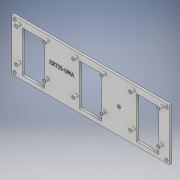
# Autodesk Inventor part: ClusterLayer3-2
Saved by Autodesk Inventor 2019 (Build 230136000, 136)
## iProperties
Created: 2019-02-04
Part Number: ClusterLayer3-2
Material: Genérico
Document SubType Name: Modeling
Designer: LuisAlonso
Density: 1 g/cm^3
Appearance: Valor por defecto
Author: LuisAlonso
Autodesk Inventor part; units mm, degrees
ref_plane "YZ Plane" through (0, 0, 0) normal (1, 0, 0) x (0, 1, 0)
ref_plane "XZ Plane" through (0, 0, 0) normal (0, 1, 0) x (-1, 0, 0)
ref_plane "XY Plane" through (0, 0, 0) normal (0, 0, 1) x (1, 0, 0)
sketch "Boceto1" plane through (0, 0, 0) normal (0, 0, 1) x (1, 0, 0)
  line L0 (0, 0) -> (275, 0)
  line L1 (275, 0) -> (275, -90)
  line L2 (275, -90) -> (0, -90)
  line L3 (0, -90) -> (0, 0)
  dimension "d0" = 275
  dimension "d1" = 90
  constraints: 8 end point, 2 perpendicular, 1 horizontal, 1 vertical
  measures "d0" distance of L0.start L0.end
  measures "d1" distance of L0.end L1.end
extrude "Extrusión1" add sketch "Boceto1" along normal blind 4
sketch "Boceto8" plane through (0, 0, 4) normal (0, 0, 1) x (1, 0, 0)
  line L0 (275, 0) -> (0, 0) projected
  line L1 (0, 0) -> (5, 0)
  line L2 (5, 0) -> (5, -5)
  circle A0 centre (5, -5) radius 1.6
  line L3 (0, 0) -> (0, -90) projected
  line L4 (0, -90) -> (5, -90)
  line L5 (5, -90) -> (5, -85)
  circle A1 centre (5, -85) radius 1.6
  line L6 (0, -90) -> (275, -90) projected
  line L7 (275, -90) -> (270, -90)
  line L8 (270, -90) -> (270, -85)
  circle A2 centre (270, -85) radius 1.6
  line L9 (275, 0) -> (270, 0)
  line L10 (270, 0) -> (270, -5)
  circle A3 centre (270, -5) radius 1.6
  dimension "d127" = 5
  dimension "d128" = 5
  dimension "d129" = 3.2
  dimension "d130" = 5
  dimension "d131" = 5
  dimension "d132" = 3.2
  dimension "d133" = 5
  dimension "d134" = 5
  dimension "d135" = 3.2
  dimension "d136" = 5
  dimension "d137" = 5
  dimension "d138" = 3.2
  constraints: 16 end point, 4 centre point, 4 coincident, 4 perpendicular, 3 point on line, 1 horizontal
  measures "d127" distance of L0.end L1.end
  measures "d128" distance of L1.end L2.end
  measures "d129" diameter of A0
  measures "d130" distance of L3.end L4.end
  measures "d131" distance of L4.end L5.end
  measures "d132" diameter of A1
  measures "d133" distance of L6.end L7.end
  measures "d134" distance of L7.end L8.end
  measures "d135" diameter of A2
  measures "d136" distance of L0.start L9.end
  measures "d137" distance of L9.end L10.end
  measures "d138" diameter of A3
extrude "Extrusión7" cut sketch "Boceto8" against normal blind 15
sketch "Boceto9" plane through (0, 0, 4) normal (0, 0, 1) x (1, 0, 0)
  line L0 (0, 0) -> (13.5, 0)
  line L1 (0, 0) -> (275, 0) projected
  line L2 (13.5, 0) -> (13.5, -8)
  circle A0 centre (13.5, -8) radius 1.5
  line L3 (13.5, -8) -> (62.5, -8)
  line L4 (13.5, -8) -> (13.5, -66)
  line L5 (62.5, -8) -> (62.5, -66)
  circle A1 centre (62.5, -8) radius 1.5
  circle A2 centre (62.5, -66) radius 1.5
  circle A3 centre (13.5, -66) radius 1.5
  dimension "d141" = 13.5
  dimension "d142" = 8
  dimension "d143" = 3
  dimension "d144" = 49
  dimension "d145" = 58
  dimension "d146" = 58
  dimension "d147" = 3
  dimension "d148" = 3
  dimension "d149" = 3
  constraints: 10 end point, 4 centre point, 4 coincident, 2 vertical, 1 horizontal, 1 perpendicular, 1 point on line
  measures "d141" distance of L0.start L0.end
  measures "d142" distance of L0.end L2.end
  measures "d143" diameter of A0
  measures "d144" distance of L3.start L3.end
  measures "d145" distance of L3.start L4.end
  measures "d146" distance of L3.end L5.end
  measures "d147" diameter of A1
  measures "d148" diameter of A2
  measures "d149" diameter of A3
extrude "Extrusión8" cut sketch "Boceto9" against normal blind 15
sketch "Boceto10" plane through (0, 0, 4) normal (0, 0, 1) x (1, 0, 0)
  line L0 (0, 0) -> (275, 0) projected
  line L1 (275, 0) -> (261.5, 0)
  line L2 (261.5, 0) -> (261.5, -8)
  circle A0 centre (261.5, -8) radius 1.5
  line L3 (261.5, -8) -> (261.5, -66)
  line L4 (261.5, -66) -> (212.5, -66)
  line L5 (212.5, -66) -> (212.5, -8)
  circle A1 centre (212.5, -8) radius 1.5
  circle A2 centre (212.5, -66) radius 1.5
  circle A3 centre (261.5, -66) radius 1.5
  dimension "d152" = 13.5
  dimension "d153" = 8
  dimension "d154" = 3
  dimension "d155" = 58
  dimension "d156" = 49
  dimension "d157" = 3
  dimension "d158" = 3
  dimension "d159" = 3
  constraints: 10 end point, 4 centre point, 4 coincident, 3 perpendicular, 1 point on line, 1 vertical
  measures "d152" distance of L0.end L1.end
  measures "d153" distance of L1.end L2.end
  measures "d154" diameter of A0
  measures "d155" distance of L3.start L3.end
  measures "d156" distance of L3.end L4.end
  measures "d157" diameter of A1
  measures "d158" diameter of A2
  measures "d159" diameter of A3
extrude "Extrusión9" cut sketch "Boceto10" against normal blind 15
sketch "Boceto11" plane through (0, 0, 4) normal (0, 0, 1) x (1, 0, 0)
  line L0 (0, 0) -> (113, 0)
  line L1 (0, 0) -> (275, 0) projected
  line L2 (113, 0) -> (113, -8)
  circle A0 centre (113, -8) radius 1.5
  line L3 (113, -8) -> (162, -8)
  line L4 (162, -8) -> (162, -66)
  line L5 (162, -66) -> (113, -66)
  circle A1 centre (113, -66) radius 1.5
  circle A2 centre (162, -66) radius 1.5
  circle A3 centre (162, -8) radius 1.5
  dimension "d162" = 113
  dimension "d163" = 8
  dimension "d164" = 3
  dimension "d165" = 49
  dimension "d166" = 58
  dimension "d167" = 3
  dimension "d168" = 3
  dimension "d169" = 3
  constraints: 10 end point, 4 centre point, 4 coincident, 3 perpendicular, 1 horizontal, 1 point on line
  measures "d162" distance of L0.start L0.end
  measures "d163" distance of L0.end L2.end
  measures "d164" diameter of A0
  measures "d165" distance of L3.start L3.end
  measures "d166" distance of L3.end L4.end
  measures "d167" diameter of A1
  measures "d168" diameter of A2
  measures "d169" diameter of A3
extrude "Extrusión10" cut sketch "Boceto11" against normal blind 15
sketch "Boceto12" plane through (0, 0, 4) normal (0, 0, 1) x (1, 0, 0)
  line L0 (275, -90) -> (0, -90) projected
  line L1 (275, -90) -> (187.25, -90)
  line L2 (187.25, -90) -> (187.25, -46)
  circle A0 centre (187.25, -46) radius 1.6
  point P0 (0, 0)
  dimension "d172" = 87.75
  dimension "d173" = 44
  dimension "d174" = 3.2
  constraints: 4 end point, 1 centre point, 1 coincident, 1 point on line, 1 vertical
  measures "d172" distance of L0.start L1.end
  measures "d173" distance of L1.end L2.end
  measures "d174" diameter of A0
extrude "Extrusión11" cut sketch "Boceto12" against normal blind 15
sketch "Boceto13" plane through (0, 0, 4) normal (0, 0, 1) x (1, 0, 0)
  line L0 (0, -90) -> (0, 0) projected
  line L1 (0, 0) -> (18.5, 0)
  line L2 (0, 0) -> (275, 0) projected
  line L3 (18.5, 0) -> (18.5, -11)
  line L4 (18.5, -11) -> (57.5, -11)
  line L5 (57.5, -11) -> (57.5, -83)
  line L6 (57.5, -83) -> (18.5, -83)
  line L7 (18.5, -83) -> (18.5, -11)
  dimension "d177" = 18.5
  dimension "d178" = 11
  dimension "d179" = 39
  dimension "d180" = 72
  dimension "d181" = 39
  constraints: 12 end point, 2 horizontal, 2 perpendicular, 1 point on line
  measures "d177" distance of L0.end L1.end
  measures "d178" distance of L1.end L3.end
  measures "d179" distance of L3.end L4.end
  measures "d180" distance of L4.end L5.end
  measures "d181" distance of L5.end L6.end
extrude "Extrusión12" cut sketch "Boceto13" against normal blind 15
sketch "Boceto14" plane through (0, 0, 4) normal (0, 0, 1) x (1, 0, 0)
  line L0 (275, 0) -> (275, -90) projected
  line L1 (275, 0) -> (256.5, 0)
  line L2 (0, 0) -> (275, 0) projected
  line L3 (256.5, 0) -> (256.5, -11)
  line L4 (256.5, -11) -> (217.5, -11)
  line L5 (217.5, -11) -> (217.5, -83)
  line L6 (217.5, -83) -> (256.5, -83)
  line L7 (256.5, -83) -> (256.5, -11)
  dimension "d184" = 18.5
  dimension "d185" = 11
  dimension "d186" = 39
  dimension "d187" = 72
  dimension "d188" = 39
  constraints: 12 end point, 3 perpendicular, 2 point on line
  measures "d184" distance of L0.start L1.end
  measures "d185" distance of L1.end L3.end
  measures "d186" distance of L3.end L4.end
  measures "d187" distance of L4.end L5.end
  measures "d188" distance of L5.end L6.end
extrude "Extrusión13" cut sketch "Boceto14" against normal blind 15
sketch "Boceto15" plane through (0, 0, 4) normal (0, 0, 1) x (1, 0, 0)
  line L0 (0, 0) -> (275, 0) projected
  line L1 (0, 0) -> (118, 0)
  line L2 (118, 0) -> (118, -11)
  line L3 (118, -11) -> (157, -11)
  line L4 (157, -11) -> (157, -83)
  line L5 (157, -83) -> (118, -83)
  line L6 (118, -83) -> (118, -11)
  dimension "d191" = 118
  dimension "d192" = 11
  dimension "d193" = 39
  dimension "d194" = 72
  dimension "d195" = 39
  constraints: 12 end point, 2 horizontal, 2 perpendicular, 1 point on line
  measures "d191" distance of L0.start L1.end
  measures "d192" distance of L1.end L2.end
  measures "d193" distance of L2.end L3.end
  measures "d194" distance of L3.end L4.end
  measures "d195" distance of L4.end L5.end
extrude "Extrusión14" cut sketch "Boceto15" against normal blind 15
sketch "Boceto17" plane through (0, 0, 4) normal (0, 0, 1) x (1, 0, 0)
  circle A0 centre (5, -5) radius 1.6 projected
  circle A1 centre (5, -5) radius 3
  circle A2 centre (13.5, -8) radius 1.5 projected
  circle A3 centre (13.5, -8) radius 3
  circle A4 centre (62.5, -8) radius 1.5 projected
  circle A5 centre (62.5, -8) radius 3
  circle A6 centre (62.5, -66) radius 1.5 projected
  circle A7 centre (62.5, -66) radius 3
  circle A8 centre (13.5, -66) radius 1.5 projected
  circle A9 centre (13.5, -66) radius 3
  circle A10 centre (5, -85) radius 1.6 projected
  circle A11 centre (5, -85) radius 3
  circle A12 centre (113, -8) radius 1.5 projected
  circle A13 centre (113, -8) radius 3
  circle A14 centre (162, -8) radius 1.5 projected
  circle A15 centre (162, -8) radius 3
  circle A16 centre (113, -66) radius 1.5 projected
  circle A17 centre (113, -66) radius 3
  circle A18 centre (162, -66) radius 1.5 projected
  circle A19 centre (162, -66) radius 3
  circle A20 centre (187.25, -46) radius 1.6 projected
  circle A21 centre (187.25, -46) radius 3
  circle A22 centre (212.5, -8) radius 1.5 projected
  circle A23 centre (212.5, -8) radius 3
  circle A24 centre (212.5, -66) radius 1.5 projected
  circle A25 centre (212.5, -66) radius 3
  circle A26 centre (261.5, -8) radius 1.5 projected
  circle A27 centre (261.5, -8) radius 3
  circle A28 centre (270, -5) radius 1.6 projected
  circle A29 centre (270, -5) radius 3
  circle A30 centre (261.5, -66) radius 1.5 projected
  circle A31 centre (261.5, -66) radius 3
  circle A32 centre (270, -85) radius 1.6 projected
  circle A33 centre (270, -85) radius 3
  circle A34 centre (62.5, -66) radius 2
  circle A35 centre (113, -8) radius 2
  circle A36 centre (162, -8) radius 2
  circle A37 centre (212.5, -8) radius 2
  circle A38 centre (212.5, -66) radius 2
  circle A39 centre (162, -66) radius 2
  circle A40 centre (113, -66) radius 2
  circle A41 centre (261.5, -8) radius 2
  circle A42 centre (261.5, -66) radius 2
  circle A43 centre (62.5, -8) radius 1.5 projected
  circle A44 centre (62.5, -8) radius 2
  circle A45 centre (13.5, -8) radius 2
  circle A46 centre (13.5, -66) radius 2
  point P0 (0, 0)
  dimension "d198" = 6
  dimension "d199" = 6
  dimension "d200" = 6
  dimension "d201" = 6
  dimension "d202" = 6
  dimension "d203" = 6
  dimension "d204" = 6
  dimension "d205" = 6
  dimension "d206" = 6
  dimension "d207" = 6
  dimension "d208" = 6
  dimension "d209" = 6
  dimension "d210" = 6
  dimension "d211" = 6
  dimension "d212" = 6
  dimension "d213" = 6
  dimension "d214" = 6
  dimension "d232" = 4
  dimension "d233" = 4
  dimension "d234" = 4
  dimension "d235" = 4
  dimension "d236" = 4
  dimension "d237" = 4
  dimension "d238" = 4
  dimension "d239" = 4
  dimension "d240" = 4
  dimension "d241" = 4
  dimension "d242" = 4
  dimension "d243" = 4
  constraints: 29 centre point, 29 coincident
  measures "d198" diameter of A1
  measures "d199" diameter of A3
  measures "d200" diameter of A5
  measures "d201" diameter of A7
  measures "d202" diameter of A9
  measures "d203" diameter of A11
  measures "d204" diameter of A13
  measures "d205" diameter of A15
  measures "d206" diameter of A17
  measures "d207" diameter of A19
  measures "d208" diameter of A21
  measures "d209" diameter of A23
  measures "d210" diameter of A25
  measures "d211" diameter of A27
  measures "d212" diameter of A29
  measures "d213" diameter of A31
  measures "d214" diameter of A33
  measures "d232" diameter of A34
  measures "d233" diameter of A35
  measures "d234" diameter of A36
  measures "d235" diameter of A37
  measures "d236" diameter of A38
  measures "d237" diameter of A39
  measures "d238" diameter of A40
  measures "d239" diameter of A41
  measures "d240" diameter of A42
  measures "d241" diameter of A44
  measures "d242" diameter of A45
  measures "d243" diameter of A46
sketch "Boceto24" plane through (0, 0, 4) normal (0, 0, 1) x (1, 0, 0)
  line L0 (65.986, -35.14) -> (108.7206, -35.14) construction
  line L1 (108.7206, -35.14) -> (108.7206, -41.4773) construction
  line L2 (108.7206, -41.4773) -> (65.986, -41.4773) construction
  line L3 (65.986, -41.4773) -> (65.986, -35.14) construction
  line L4 (66.6039, -41.3488) -> (66.6039, -35.2488)
  line L5 (66.6039, -35.2488) -> (70.4201, -35.2488)
  line L6 (70.4201, -35.2488) -> (70.4201, -35.9705)
  line L7 (70.4201, -35.9705) -> (67.4146, -35.9705)
  line L8 (67.4146, -35.9705) -> (67.4146, -37.6413)
  line L9 (67.4146, -37.6413) -> (70.2174, -37.6413)
  line L10 (70.2174, -37.6413) -> (70.2174, -38.363)
  line L11 (70.2174, -38.363) -> (67.4146, -38.363)
  line L12 (67.4146, -38.363) -> (67.4146, -40.6271)
  line L13 (67.4146, -40.6271) -> (70.4201, -40.6271)
  line L14 (70.4201, -40.6271) -> (70.4201, -41.3488)
  line L15 (70.4201, -41.3488) -> (66.6039, -41.3488)
  line L16 (76.0307, -41.3488) -> (74.9778, -41.3488)
  line L17 (74.9778, -41.3488) -> (73.0499, -38.9216)
  line L18 (73.0499, -38.9216) -> (72.1206, -38.9216)
  line L19 (72.1206, -38.9216) -> (72.1206, -41.3488)
  line L20 (72.1206, -41.3488) -> (71.3099, -41.3488)
  line L21 (71.3099, -41.3488) -> (71.3099, -35.2488)
  line L22 (71.3099, -35.2488) -> (72.8819, -35.2488)
  spline S0 degree 2 poles (72.8819, -35.2488) (73.4058, -35.2488) (74.1127, -35.3625) (74.434, -35.5701) knots 0 0 0 1 2 2 2
  spline S1 degree 2 poles (74.434, -35.5701) (74.7554, -35.7777) (75.1261, -36.4253) (75.1261, -36.9048) knots 0 0 0 1 2 2 2
  spline S2 degree 2 poles (75.1261, -36.9048) (75.1261, -37.5721) (74.4439, -38.4767) (73.8606, -38.6942) knots 0 0 0 1 2 2 2
  line L23 (73.8606, -38.6942) -> (76.0307, -41.3488)
  spline S3 degree 2 poles (74.2808, -36.969) (74.2808, -36.7021) (74.093, -36.2918) (73.8952, -36.1583) knots 0 0 0 1 2 2 2
  spline S4 degree 2 poles (73.8952, -36.1583) (73.7222, -36.0446) (73.2625, -35.9507) (72.9263, -35.9507) knots 0 0 0 1 2 2 2
  line L24 (72.9263, -35.9507) -> (72.1206, -35.9507)
  line L25 (72.1206, -35.9507) -> (72.1206, -38.2444)
  line L26 (72.1206, -38.2444) -> (72.8324, -38.2444)
  spline S5 degree 2 poles (72.8324, -38.2444) (73.1834, -38.2444) (73.742, -38.1208) (73.9348, -37.928) knots 0 0 0 1 2 2 2
  spline S6 degree 2 poles (73.9348, -37.928) (74.1127, -37.76) (74.2808, -37.2854) (74.2808, -36.969) knots 0 0 0 1 2 2 2
  line L27 (77.9388, -41.3488) -> (77.9388, -35.9705)
  line L28 (77.9388, -35.9705) -> (75.8923, -35.9705)
  line L29 (75.8923, -35.9705) -> (75.8923, -35.2488)
  line L30 (75.8923, -35.2488) -> (80.796, -35.2488)
  line L31 (80.796, -35.2488) -> (80.796, -35.9705)
  line L32 (80.796, -35.9705) -> (78.7495, -35.9705)
  line L33 (78.7495, -35.9705) -> (78.7495, -41.3488)
  line L34 (78.7495, -41.3488) -> (77.9388, -41.3488)
  line L35 (83.5396, -41.3488) -> (81.1767, -41.3488)
  line L36 (81.1767, -41.3488) -> (81.1767, -40.7259)
  line L37 (81.1767, -40.7259) -> (81.9528, -40.7259)
  line L38 (81.9528, -40.7259) -> (81.9528, -35.8716)
  line L39 (81.9528, -35.8716) -> (81.1767, -35.8716)
  line L40 (81.1767, -35.8716) -> (81.1767, -35.2488)
  line L41 (81.1767, -35.2488) -> (83.5396, -35.2488)
  line L42 (83.5396, -35.2488) -> (83.5396, -35.8716)
  line L43 (83.5396, -35.8716) -> (82.7635, -35.8716)
  line L44 (82.7635, -35.8716) -> (82.7635, -40.7259)
  line L45 (82.7635, -40.7259) -> (83.5396, -40.7259)
  line L46 (83.5396, -40.7259) -> (83.5396, -41.3488)
  spline S7 degree 2 poles (86.2435, -41.4575) (85.5811, -41.4575) (84.6518, -41.1807) (84.2415, -40.983) knots 0 0 0 1 2 2 2
  line L47 (84.2415, -40.983) -> (84.2415, -39.9647)
  line L48 (84.2415, -39.9647) -> (84.3008, -39.9647)
  spline S8 degree 2 poles (84.3008, -39.9647) (84.7012, -40.3404) (85.7146, -40.7556) (86.1842, -40.7556) knots 0 0 0 1 2 2 2
  spline S9 degree 2 poles (86.1842, -40.7556) (86.8565, -40.7556) (87.5436, -40.197) (87.5436, -39.7373) knots 0 0 0 1 2 2 2
  spline S10 degree 2 poles (87.5436, -39.7373) (87.5436, -39.3715) (87.1828, -38.9167) (86.7922, -38.803) knots 0 0 0 1 2 2 2
  spline S11 degree 2 poles (86.7922, -38.803) (86.5105, -38.7239) (86.0409, -38.6151) (85.6899, -38.5262) knots 0 0 0 1 2 2 2
  spline S12 degree 2 poles (85.6899, -38.5262) (85.3735, -38.4421) (84.8742, -38.19) (84.6815, -37.9874) knots 0 0 0 1 2 2 2
  spline S13 degree 2 poles (84.6815, -37.9874) (84.4936, -37.7847) (84.286, -37.2409) (84.286, -36.885) knots 0 0 0 1 2 2 2
  spline S14 degree 2 poles (84.286, -36.885) (84.286, -36.1435) (85.4427, -35.14) (86.3375, -35.14) knots 0 0 0 1 2 2 2
  spline S15 degree 2 poles (86.3375, -35.14) (86.8516, -35.14) (87.7611, -35.3427) (88.1516, -35.5355) knots 0 0 0 1 2 2 2
  line L49 (88.1516, -35.5355) -> (88.1516, -36.5044)
  line L50 (88.1516, -36.5044) -> (88.0923, -36.5044)
  spline S16 degree 2 poles (88.0923, -36.5044) (87.8007, -36.2374) (86.8911, -35.842) (86.3918, -35.842) knots 0 0 0 1 2 2 2
  spline S17 degree 2 poles (86.3918, -35.842) (85.8283, -35.842) (85.1313, -36.3709) (85.1313, -36.801) knots 0 0 0 1 2 2 2
  spline S18 degree 2 poles (85.1313, -36.801) (85.1313, -37.1865) (85.5416, -37.6463) (85.9272, -37.7501) knots 0 0 0 1 2 2 2
  spline S19 degree 2 poles (85.9272, -37.7501) (86.1842, -37.8193) (86.9306, -37.9972) (87.1778, -38.0714) knots 0 0 0 1 2 2 2
  spline S20 degree 2 poles (87.1778, -38.0714) (87.8056, -38.2642) (88.3889, -39.0403) (88.3889, -39.6087) knots 0 0 0 1 2 2 2
  spline S21 degree 2 poles (88.3889, -39.6087) (88.3889, -39.9696) (88.0973, -40.6617) (87.8353, -40.9039) knots 0 0 0 1 2 2 2
  spline S22 degree 2 poles (87.8353, -40.9039) (87.5436, -41.1708) (86.8021, -41.4575) (86.2435, -41.4575) knots 0 0 0 1 2 2 2
  line L51 (91.2758, -39.0502) -> (88.9673, -39.0502)
  line L52 (88.9673, -39.0502) -> (88.9673, -38.3087)
  line L53 (88.9673, -38.3087) -> (91.2758, -38.3087)
  line L54 (91.2758, -38.3087) -> (91.2758, -39.0502)
  spline S23 degree 2 poles (94.39, -41.4773) (93.8512, -41.4773) (93.0504, -41.1955) (92.7687, -40.9138) knots 0 0 0 1 2 2 2
  spline S24 degree 2 poles (92.7687, -40.9138) (92.4473, -40.5974) (92.1853, -39.7076) (92.1853, -39.0551) knots 0 0 0 1 2 2 2
  line L55 (92.1853, -39.0551) -> (92.1853, -35.2488)
  line L56 (92.1853, -35.2488) -> (92.996, -35.2488)
  line L57 (92.996, -35.2488) -> (92.996, -39.0551)
  spline S25 degree 2 poles (92.996, -39.0551) (92.996, -39.4802) (93.1048, -40.0536) (93.258, -40.286) knots 0 0 0 1 2 2 2
  spline S26 degree 2 poles (93.258, -40.286) (93.4212, -40.5331) (93.9847, -40.7852) (94.39, -40.7852) knots 0 0 0 1 2 2 2
  spline S27 degree 2 poles (94.39, -40.7852) (94.7707, -40.7852) (95.3639, -40.5331) (95.527, -40.286) knots 0 0 0 1 2 2 2
  spline S28 degree 2 poles (95.527, -40.286) (95.6802, -40.0536) (95.789, -39.4852) (95.789, -39.0749) knots 0 0 0 1 2 2 2
  line L58 (95.789, -39.0749) -> (95.789, -35.2488)
  line L59 (95.789, -35.2488) -> (96.5997, -35.2488)
  line L60 (96.5997, -35.2488) -> (96.5997, -39.0551)
  spline S29 degree 2 poles (96.5997, -39.0551) (96.5997, -39.6928) (96.3426, -40.6023) (96.0164, -40.9138) knots 0 0 0 1 2 2 2
  spline S30 degree 2 poles (96.0164, -40.9138) (95.7247, -41.2005) (94.9536, -41.4773) (94.39, -41.4773) knots 0 0 0 1 2 2 2
  line L61 (102.9913, -41.3488) -> (102.1806, -41.3488)
  line L62 (102.1806, -41.3488) -> (102.1806, -36.0941)
  line L63 (102.1806, -36.0941) -> (100.5889, -39.6681)
  line L64 (100.5889, -39.6681) -> (100.0946, -39.6681)
  line L65 (100.0946, -39.6681) -> (98.5177, -36.0941)
  line L66 (98.5177, -36.0941) -> (98.5177, -41.3488)
  line L67 (98.5177, -41.3488) -> (97.7614, -41.3488)
  line L68 (97.7614, -41.3488) -> (97.7614, -35.2488)
  line L69 (97.7614, -35.2488) -> (98.8687, -35.2488)
  line L70 (98.8687, -35.2488) -> (100.3912, -38.6448)
  line L71 (100.3912, -38.6448) -> (101.8643, -35.2488)
  line L72 (101.8643, -35.2488) -> (102.9913, -35.2488)
  line L73 (102.9913, -35.2488) -> (102.9913, -41.3488)
  line L74 (103.5697, -41.3488) -> (105.6261, -35.2488)
  line L75 (105.6261, -35.2488) -> (106.6246, -35.2488)
  line L76 (106.6246, -35.2488) -> (108.681, -41.3488)
  line L77 (108.681, -41.3488) -> (107.8259, -41.3488)
  line L78 (107.8259, -41.3488) -> (107.2722, -39.6433)
  line L79 (107.2722, -39.6433) -> (104.9439, -39.6433)
  line L80 (104.9439, -39.6433) -> (104.3903, -41.3488)
  line L81 (104.3903, -41.3488) -> (103.5697, -41.3488)
  line L82 (107.0498, -38.9513) -> (106.1056, -36.0792)
  line L83 (106.1056, -36.0792) -> (105.1664, -38.9513)
  line L84 (105.1664, -38.9513) -> (107.0498, -38.9513)
  point P0 (0, 0)
  constraints: 2 other
extrude "Extrusión17" cut sketch "Boceto24" against normal blind 10
sketch "Boceto26" plane through (0, 0, 4) normal (0, 0, 1) x (1, 0, 0)
  circle A0 centre (5, -5) radius 1.6 projected
  circle A1 centre (5, -5) radius 3
  circle A2 centre (270, -85) radius 1.6 projected
  circle A3 centre (270, -85) radius 3
  circle A4 centre (270, -5) radius 1.6 projected
  circle A5 centre (270, -5) radius 3
  circle A6 centre (5, -85) radius 1.6 projected
  circle A7 centre (5, -85) radius 3
  circle A8 centre (187.25, -46) radius 1.6 projected
  circle A9 centre (187.25, -46) radius 3
  point P0 (0, 0)
  dimension "d223" = 6
  dimension "d224" = 6
  dimension "d225" = 6
  dimension "d226" = 6
  dimension "d227" = 6
  constraints: 5 centre point, 5 coincident
  measures "d223" diameter of A1
  measures "d224" diameter of A3
  measures "d225" diameter of A5
  measures "d226" diameter of A7
  measures "d227" diameter of A9
extrude "Extrusión19" add sketch "Boceto26" along normal blind 0.2
extrude "Extrusión21" add sketch "Boceto17" along normal blind 6 contours A3 | A5 | A7 | A9 | A13 | A15 | A17 | A19 | A23 | A25 | A27 | A31
